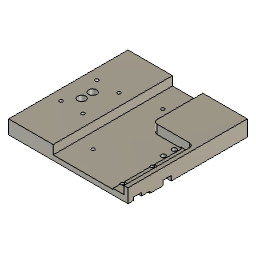
y_stage (Autodesk Fusion 360 design; units mm, degrees)
part number: 2025-09-14-19-37-15-685
Autodesk Fusion 360 part; units mm, degrees
sketch "Sketch1" plane through (0, 0, 0) normal (0, 0, 1) x (1, 0, 0)
  line L0 (-30, 30) -> (30, 30)
  line L1 (30, -30) -> (-30, -30)
  line L2 (-30, -30) -> (-30, 30)
  line L3 (-30, 30) -> (30, -30) construction
  line L4 (30, 30) -> (-30, -30) construction
  line L5 (30, -30) -> (30, 30)
  dimension "d1" = 60
  dimension "d2" = 60
  constraint horizontal L0
  constraint parallel L0 L1
  constraint coincident L3 origin
  constraint coincident L4 origin
  constraint vertical L5
  constraint horizontal L1.start L3.end
  constraint coincident L1.start L3.end
  constraint vertical L2
  measures "d1" distance of L0.start L0.end
  measures "d2" distance of L0.start L1.end
extrude "Extrude1" add sketch "Sketch1" along normal blind 8
sketch "Sketch2" plane through (0, 0, 8) normal (0, 0, 1) x (-1, 0, 0)
  line L0 (30, 30) -> (-30, 30)
  line L1 (-30, 30) -> (-30, -30)
  line L2 (-30, -30) -> (30, -30)
  line L3 (30, -30) -> (30, 30)
  line L4 (7.6, -30) -> (-7.6, -30)
  line L5 (-7.6, -30) -> (-7.6, 30)
  line L6 (-7.6, 30) -> (7.6, 30)
  line L7 (7.6, 30) -> (7.6, -30)
  line L8 (7.6, -30) -> (-7.6, 30) construction
  line L9 (-7.6, -30) -> (7.6, 30) construction
  line L10 (-7.6, 30) -> (-28, 30)
  line L11 (-28, 30) -> (-28, -5)
  line L12 (-28, -5) -> (-7.6, -5)
  line L13 (-7.6, -5) -> (-7.6, 30)
  dimension "d6" = 15.2
  dimension "d23" = 35
  dimension "d24" = 20.4
  constraint horizontal L4
  constraint perpendicular L4 L5
  constraint parallel L4 L6
  constraint parallel L5 L7
  constraint coincident L8 origin
  constraint coincident L9 origin
  constraint coincident L2 L4.start
  constraint horizontal L10
  constraint vertical L11
  constraint horizontal L12
  constraint vertical L13
  measures "d6" distance of L4.start L4.end
  measures "d23" distance of L10.end L11.end
  measures "d24" distance of L11.end L12.end
extrude "Extrude2" cut sketch "Sketch2" against normal blind 4.5 contours L0 L2 L4 L5 L6 L7 L13 | L0 L5 L10 L11 L12 L13
sketch "Sketch3" plane through (0, 0, 8) normal (0, 0, 1) x (-1, 0, 0)
  line L0 (7.6, 30) -> (-7.6, 30)
  line L1 (-7.6, 30) -> (-7.6, -30)
  line L2 (-7.6, -30) -> (7.6, -30)
  line L3 (7.6, -30) -> (7.6, 30)
  circle A0 centre (0, -17.5) radius 1.5
  circle A1 centre (0, 17.5) radius 1.5
  line L4 (7.6, 30) -> (7.6, -30)
  line L5 (7.6, -30) -> (30, -30)
  line L6 (30, -30) -> (30, 30)
  line L7 (30, 30) -> (7.6, 30)
  circle A2 centre (20.5, -2.75) radius 1.125
  circle A3 centre (20.5, 2.75) radius 1.125
  circle A4 centre (-20.5, 2.75) radius 1.125
  circle A5 centre (-20.5, -2.75) radius 1.125
  line L8 (-22.5, 11.2805) -> (-26.5, 11.2805)
  arc A6 (-26.5, 11.2805) -> (-26.5, 9.2805) centre (-26.5, 10.2805) ccw
  line L9 (-26.5, 9.2805) -> (-22.5, 9.2805)
  arc A7 (-22.5, 9.2805) -> (-22.5, 11.2805) centre (-22.5, 10.2805) ccw
  line L10 (-22.5, 10.2805) -> (-26.5, 10.2805) construction
  line L11 (-22.5, 26.2805) -> (-26.5, 26.2805)
  arc A8 (-26.5, 26.2805) -> (-26.5, 24.2805) centre (-26.5, 25.2805) ccw
  line L12 (-26.5, 24.2805) -> (-22.5, 24.2805)
  arc A9 (-22.5, 24.2805) -> (-22.5, 26.2805) centre (-22.5, 25.2805) ccw
  line L13 (-22.5, 25.2805) -> (-26.5, 25.2805) construction
  line L14 (-30, 30) -> (-30, -30)
  line L15 (-28, 30) -> (7.6, 30)
  circle A10 centre (13.6, 9) radius 1.5
  circle A11 centre (24.6, 9) radius 1.5
  circle A12 centre (13.6, -9) radius 1.5
  circle A13 centre (24.6, -9) radius 1.5
  dimension "d9" = 3
  dimension "d10" = 35
  dimension "d11" = 17.5
  dimension "d14" = 2.25
  dimension "d15" = 41
  dimension "d16" = 5.5
  dimension "d17" = 2.75
  dimension "d18" = 20.5
  dimension "d28" = 15
  dimension "d29" = 1
  dimension "d30" = 4
  dimension "d31" = 7.5
  dimension "d36" = 4.7195
  dimension "d60" = 3
  dimension "d61" = 18
  dimension "d62" = 11
  dimension "d63" = 21
  dimension "d64" = 6
  constraint equal A0 A1
  constraint vertical origin A0.centre
  constraint vertical origin A1.centre
  constraint vertical A2.centre A3.centre
  constraint horizontal A3.centre A4.centre
  constraint vertical A4.centre A5.centre
  constraint horizontal A2.centre A5.centre
  constraint equal A4 A5
  constraint equal A2 A5
  constraint equal A2 A3
  constraint tangent L8 A6
  constraint tangent A6 L9
  constraint parallel L8 L9
  constraint tangent L9 A7
  constraint tangent L8 A7
  constraint horizontal L10
  constraint tangent L11 A8
  constraint tangent A8 L12
  constraint parallel L11 L12
  constraint tangent L12 A9
  constraint tangent L11 A9
  constraint horizontal L13
  constraint vertical A7.centre A9.centre
  constraint vertical A6.centre A8.centre
  constraint equal A7 A9
  constraint horizontal A10.centre A11.centre
  constraint vertical A11.centre A13.centre
  constraint horizontal A12.centre A13.centre
  constraint vertical A10.centre A12.centre
  constraint equal A10 A12
  constraint equal A12 A13
  constraint equal A10 A11
  measures "d9" diameter of A1
  measures "d10" distance of A0.centre A1.centre
  measures "d11" distance of origin A0.centre
  measures "d14" diameter of A2
  measures "d15" distance of A2.centre A5.centre
  measures "d16" distance of A2.centre A3.centre
  measures "d17" vertical distance of origin A3.centre
  measures "d18" horizontal distance of origin A2.centre
  measures "d28" distance of A6.centre A8.centre
  measures "d29" distance of A7 L10
  measures "d30" distance of A6.end L9.end
  measures "d31" distance of A7.centre L14
  measures "d36" distance of A9.centre L15
  measures "d60" diameter of A10
  measures "d61" distance of A10.centre A12.centre
  measures "d62" distance of A10.centre A11.centre
  measures "d63" distance of L7 A11.centre
  measures "d64" distance of L3 A10.centre
extrude "Extrude3" cut sketch "Sketch3" against normal up to surface (8 mm away) contours A0 | A1 | A2 | A3 | A4 | A5 | L8 A6 L9 A7 | L11 A8 L12 A9 | A10 | A11 | A12 | A13
sketch "Sketch4" plane through (0, 0, 3.5) normal (0, 0, 1) x (-1, 0, 0)
  circle A0 centre (0, -17.5) radius 1.5
  circle A1 centre (-20.5, -2.75) radius 1.125
  circle A2 centre (0, 17.5) radius 1.5
  circle A3 centre (-20.5, 2.75) radius 1.125
  line L0 (7.6, 30) -> (-28, 30)
  line L1 (-28, 30) -> (-28, -5)
  line L2 (-28, -5) -> (-7.6, -5)
  line L3 (-7.6, -5) -> (-7.6, -30)
  line L4 (-7.6, -30) -> (7.6, -30)
  line L5 (7.6, -30) -> (7.6, 30)
  line L6 (-28, -5) -> (-22.5, -5)
  line L7 (-22.5, -5) -> (-22.5, 30)
  line L8 (-22.5, 30) -> (-28, 30)
  line L9 (-28, 30) -> (-28, -5)
  line L10 (-22.5, 24.2805) -> (-26.5, 24.2805)
  line L11 (-26.5, 26.2805) -> (-22.5, 26.2805)
  arc A4 (-22.5, 24.2805) -> (-22.5, 26.2805) centre (-22.5, 25.2805) ccw
  line L12 (-22.5, 9.2805) -> (-26.5, 9.2805)
  line L13 (-26.5, 11.2805) -> (-22.5, 11.2805)
  arc A5 (-22.5, 9.2805) -> (-22.5, 11.2805) centre (-22.5, 10.2805) ccw
  arc A6 (-26.5, 26.2805) -> (-26.5, 24.2805) centre (-26.5, 25.2805) ccw
  arc A7 (-26.5, 11.2805) -> (-26.5, 9.2805) centre (-26.5, 10.2805) ccw
  dimension "d25" = 5.5
  constraint horizontal L6
  constraint vertical L7
  constraint horizontal L8
  constraint vertical L9
  constraint coincident L0 L7.end
  constraint coincident L1.end L2.start
  measures "d25" distance of L7.end L0.end
extrude "Extrude4" add sketch "Sketch4" along normal blind 0.5 contours L0 L1 L2 L6 L7 L8 L9 L10 L11 L12 L13 A6 A7
fillet "Fillet1" radius 2 2 edges at (7.6, 5, 5.75) (28, 5, 6)
fillet "Fillet2" radius 1 1 edges at (22.5, 5, 3.75)
sketch "Sketch5" plane through (0, 0, 0) normal (0, 0, -1) x (1, 0, 0)
  circle A0 centre (20.5, 2.75) radius 1.125
  circle A1 centre (0, 17.5) radius 1
  circle A2 centre (-20.5, -2.75) radius 1.125
  line L0 (26.5, 24.2805) -> (22.5, 24.2805)
  arc A3 (22.5, 26.2805) -> (22.5, 24.2805) centre (22.5, 25.2805) ccw
  line L1 (22.5, 26.2805) -> (26.5, 26.2805)
  arc A4 (26.5, 24.2805) -> (26.5, 26.2805) centre (26.5, 25.2805) ccw
  circle A5 centre (20.5, -2.75) radius 1.125
  circle A6 centre (0, -17.5) radius 1
  circle A7 centre (-20.5, 2.75) radius 1.125
  line L2 (26.5, 9.2805) -> (22.5, 9.2805)
  arc A8 (22.5, 11.2805) -> (22.5, 9.2805) centre (22.5, 10.2805) ccw
  line L3 (22.5, 11.2805) -> (26.5, 11.2805)
  arc A9 (26.5, 9.2805) -> (26.5, 11.2805) centre (26.5, 10.2805) ccw
  line L4 (30, 30) -> (-30, 30)
  line L5 (-30, 30) -> (-30, -30)
  line L6 (-30, -30) -> (30, -30)
  line L7 (30, -30) -> (30, 30)
  line L8 (30, -30) -> (-30, -30)
  line L9 (-30, -30) -> (-30, -19.5)
  line L10 (-30, -19.5) -> (30, -19.5)
  line L11 (30, -19.5) -> (30, -30)
  line L12 (0, 0) -> (-6.6567, 0) construction
  line L13 (-30, 30) -> (-30, 19.5)
  line L14 (-30, 19.5) -> (30, 19.5)
  line L15 (30, 19.5) -> (30, 30)
  line L16 (30, 30) -> (-30, 30)
  circle A10 centre (-13.6, 9) radius 1
  circle A11 centre (-24.6, 9) radius 1
  circle A12 centre (-13.6, -9) radius 1
  circle A13 centre (-24.6, -9) radius 1
  dimension "d49" = 10.5
  constraint horizontal L8
  constraint vertical L9
  constraint horizontal L10
  constraint vertical L11
  constraint coincident L5 L9.end
  constraint coincident L6.end L7.start
  constraint coincident L12.start origin
  constraint horizontal L12
  constraint symmetric L6.end L12 L4.start
  constraint symmetric L5.end L12 L4.end
  constraint symmetric L9.end L12 L13.end
  constraint symmetric L10.end L12 L14.end
  measures "d49" distance of L5.end L9.end
extrude "Extrude5" [suppressed]
sketch "Sketch6" plane through (0, 0, 0) normal (0, 0, -1) x (1, 0, 0)
  line L0 (30, -30) -> (30, 19.5)
  line L1 (-30, 19.5) -> (-30, -30)
  line L2 (26.5, 9.2805) -> (22.5, 9.2805)
  arc A0 (22.5, 11.2805) -> (22.5, 9.2805) centre (22.5, 10.2805) ccw
  line L3 (22.5, 11.2805) -> (26.5, 11.2805)
  arc A1 (26.5, 9.2805) -> (26.5, 11.2805) centre (26.5, 10.2805) ccw
  circle A2 centre (-20.5, 2.75) radius 1.125
  circle A3 centre (0, -17.5) radius 1
  circle A4 centre (20.5, -2.75) radius 1.125
  circle A5 centre (-20.5, -2.75) radius 1.125
  circle A6 centre (0, 17.5) radius 1
  circle A7 centre (20.5, 2.75) radius 1.125
  line L4 (22.5, 23.2805) -> (26.5, 23.2805)
  arc A8 (26.5, 23.2805) -> (26.5, 27.2805) centre (26.5, 25.2805) ccw
  line L5 (26.5, 27.2805) -> (22.5, 27.2805)
  arc A9 (22.5, 27.2805) -> (22.5, 23.2805) centre (22.5, 25.2805) ccw
  line L6 (22.5, 25.2805) -> (26.5, 25.2805) construction
  line L7 (22.5, 8.2805) -> (26.5, 8.2805)
  arc A10 (26.5, 8.2805) -> (26.5, 12.2805) centre (26.5, 10.2805) ccw
  line L8 (26.5, 12.2805) -> (22.5, 12.2805)
  arc A11 (22.5, 12.2805) -> (22.5, 8.2805) centre (22.5, 10.2805) ccw
  line L9 (22.5, 10.2805) -> (26.5, 10.2805) construction
  line L10 (26.5, 27.2805) -> (30, 27.2805)
  line L11 (30, 27.2805) -> (30, 23.2805)
  line L12 (30, 23.2805) -> (26.5, 23.2805)
  line L13 (26.5, 23.2805) -> (26.5, 27.2805)
  line L14 (26.5, 12.2805) -> (30, 12.2805)
  line L15 (30, 12.2805) -> (30, 8.2805)
  line L16 (30, 8.2805) -> (26.5, 8.2805)
  line L17 (26.5, 8.2805) -> (26.5, 12.2805)
  line L18 (30, 19.5) -> (-30, 19.5)
  line L19 (-30, -30) -> (30, -30)
  circle A12 centre (-13.6, -9) radius 1
  circle A13 centre (-24.6, -9) radius 1
  circle A14 centre (-13.6, 9) radius 1
  circle A15 centre (-24.6, 9) radius 1
  arc A16 (22.5, 26.2805) -> (22.5, 24.2805) centre (22.5, 25.2805) ccw
  line L20 (26.5, 26.2805) -> (22.5, 26.2805)
  arc A17 (26.5, 24.2805) -> (26.5, 26.2805) centre (26.5, 25.2805) ccw
  line L21 (22.5, 24.2805) -> (26.5, 24.2805)
  line L22 (-30, 30) -> (-30, -30)
  line L23 (-30, -30) -> (30, -30)
  line L24 (30, -30) -> (30, 30)
  circle A18 centre (-13.6, 9) radius 1.5
  circle A19 centre (20.5, 2.75) radius 1.125
  circle A20 centre (0, 17.5) radius 1.5
  circle A21 centre (-20.5, -2.75) radius 1.125
  circle A22 centre (-24.6, 9) radius 1.5
  circle A23 centre (-13.6, -9) radius 1.5
  circle A24 centre (20.5, -2.75) radius 1.125
  circle A25 centre (0, -17.5) radius 1.5
  circle A26 centre (-20.5, 2.75) radius 1.125
  line L25 (26.5, 9.2805) -> (22.5, 9.2805)
  arc A27 (22.5, 11.2805) -> (22.5, 9.2805) centre (22.5, 10.2805) ccw
  line L26 (22.5, 11.2805) -> (26.5, 11.2805)
  arc A28 (26.5, 9.2805) -> (26.5, 11.2805) centre (26.5, 10.2805) ccw
  circle A29 centre (-24.6, -9) radius 1.5
  line L27 (26.5, 24.2805) -> (22.5, 24.2805)
  arc A30 (22.5, 26.2805) -> (22.5, 24.2805) centre (22.5, 25.2805) ccw
  line L28 (22.5, 26.2805) -> (26.5, 26.2805)
  arc A31 (26.5, 24.2805) -> (26.5, 26.2805) centre (26.5, 25.2805) ccw
  line L29 (30, 30) -> (-30, 30)
  dimension "d56" = 2
  dimension "d57" = 2
  constraint tangent L4 A8
  constraint tangent A8 L5
  constraint parallel L4 L5
  constraint tangent L5 A9
  constraint tangent L4 A9
  constraint horizontal L6
  constraint tangent L7 A10
  constraint tangent A10 L8
  constraint parallel L7 L8
  constraint tangent L8 A11
  constraint tangent L7 A11
  constraint coincident A1.centre A10.centre
  constraint parallel L4 L9
  constraint coincident A0.centre A11.centre
  constraint horizontal L10
  constraint vertical L11
  constraint horizontal L12
  constraint vertical L13
  constraint coincident L0 L11.end
  constraint collinear L4 L12
  constraint horizontal L14
  constraint vertical L15
  constraint horizontal L16
  constraint vertical L17
  constraint coincident L0 L15.end
  constraint collinear L7 L16
  constraint vertical A9.centre A0.centre
  constraint coincident A9.centre L6.start
  constraint vertical A8.centre A1.centre
  measures "d56" radius of A11
  measures "d57" radius of A9
extrude "Extrude6" cut sketch "Sketch6" against normal blind 2.5 contours L0 A10 L14 L15 L16 L24 | A1 A10 L17 A28 | L2 A0 L3 L7 L8 A11 L17 L25 A27 L26 | A8 L10 L11 L12 L24 | A8 L13 A17 A31 | L4 L5 A9 L13 A16 L20 L21 L27 A30 L28 | L13 A16 L20 L21 L27 A30 L28 | L13 A17 A31
sketch "Sketch7" plane through (0, 0, 8) normal (0, 0, 1) x (-1, 0, 0)
  circle A0 centre (13.6, 9) radius 1.5
  circle A1 centre (20.5, -2.75) radius 1.125
  circle A2 centre (24.6, 9) radius 1.5
  circle A3 centre (13.6, -9) radius 1.5
  circle A4 centre (20.5, 2.75) radius 1.125
  circle A5 centre (24.6, -9) radius 1.5
  line L0 (7.6, 30) -> (7.6, -30)
  line L1 (7.6, -30) -> (30, -30)
  line L2 (30, -30) -> (30, 30)
  line L3 (30, 30) -> (7.6, 30)
  circle A6 centre (20.5, 2.75) radius 1.125
  circle A7 centre (20.5, -2.75) radius 1.125
  circle A8 centre (20.5, 2.75) radius 2
  circle A9 centre (20.5, -2.75) radius 2
  dimension "d69" = 4
  dimension "d70" = 4
  constraint concentric A6 A8
  constraint concentric A7 A9
  measures "d69" diameter of A9
  measures "d70" diameter of A8
extrude "Extrude7" cut sketch "Sketch7" against normal up to surface (4.5 mm away) contours A8 | A9
sketch "Sketch8" plane through (-30, 0, 0) normal (-1, 0, 0) x (0, -1, 0)
  line L0 (19.5, 0) -> (19.5, 0.75)
  line L1 (19.5, 0.75) -> (30, 0.75)
  line L2 (30, 0.75) -> (30, 8)
  line L3 (30, 8) -> (-30, 8)
  line L4 (-30, 8) -> (-30, 0)
  line L5 (-30, 0) -> (19.5, 0)
  line L6 (-30, 0) -> (-22, 0)
  line L7 (-22, 0) -> (-22, 1.5)
  line L8 (-22, 1.5) -> (-30, 1.5)
  line L9 (-30, 1.5) -> (-30, 0)
  dimension "d73" = 1.5
  dimension "d74" = 8
  constraint horizontal L6
  constraint vertical L7
  constraint horizontal L8
  constraint vertical L9
  constraint coincident L4.end L5.start
  measures "d73" distance of L4.end L8.end
  measures "d74" distance of L7.end L8.end
extrude "Extrude8" [suppressed]
thread "Thread2" "ISO Metric profile 2.0 M2x0.4 M2x0.4 6H" major diameter 2.074 minor diameter 1.623 pitch 0.4 angle 60 resizes the face on face at (-1.4925, -17.3506, 2.3333) on face at (-1.4925, 17.6494, 2.3333) on face at (-26.0925, -8.8506, 2.6667) on face at (-15.0925, -8.8506, 2.6667) on face at (-26.0925, 9.1494, 2.6667) on face at (-15.0925, 9.1494, 2.6667)
sketch "Sketch10" plane through (-30, 0, 0) normal (-1, 0, 0) x (0, -1, 0)
  line L0 (-30, 0) -> (30, 0)
  line L1 (30, 0) -> (30, 8)
  line L2 (30, 8) -> (-30, 8)
  line L3 (-30, 8) -> (-30, 0)
  line L4 (30, 0) -> (19, 0)
  line L5 (19, 0) -> (19, 1)
  line L6 (19, 1) -> (30, 1)
  line L7 (30, 1) -> (30, 0)
  dimension "d88" = 1
  dimension "d90" = 11
  dimension "d97" = 49
  constraint horizontal L4
  constraint vertical L5
  constraint horizontal L6
  constraint vertical L7
  constraint coincident L0 L1.start
  measures "d88" distance of L0.end L6.end
  measures "d90" distance of L5.end L6.end
  measures "d97" distance of L0.start L4.end
extrude "Extrude10" cut sketch "Sketch10" against normal up to surface (60 mm away) contours L0 L1 L4 L5 L6 L7
sketch "Sketch9" plane through (0, 0, 8) normal (0, 0, 1) x (-1, 0, 0)
  circle A0 centre (20.28, -2.75) radius 2
  circle A1 centre (20.28, 2.75) radius 2
  circle A2 centre (13.6, 9) radius 1.5
  circle A3 centre (24.6, 9) radius 1.5
  circle A4 centre (13.6, -9) radius 1.5
  circle A5 centre (24.6, -9) radius 1.5
  line L0 (7.6, 30) -> (7.6, -30)
  line L1 (7.6, -30) -> (30, -30)
  line L2 (30, -30) -> (30, 30)
  line L3 (30, 30) -> (7.6, 30)
  line L4 (39.6, 11) -> (11.6, 11)
  line L5 (11.6, 11) -> (11.6, -11)
  line L6 (11.6, -11) -> (39.6, -11)
  line L7 (10.45, 12.5) -> (30, 12.5)
  line L8 (30, 12.5) -> (30, -12.5)
  line L9 (30, -12.5) -> (10.45, -12.5)
  line L10 (10.45, -12.5) -> (10.45, 12.5)
  dimension "d77" = 1.15
  dimension "d78" = 1.5
  dimension "d79" = 1.5
  constraint horizontal L7
  constraint vertical L8
  constraint horizontal L9
  constraint vertical L10
  constraint coincident L2 L8.end
  measures "d77" distance of L5 L10
  measures "d78" distance of L4 L7
  measures "d79" distance of L6 L9
extrude "Extrude9" [suppressed]
fillet "Fillet3" [suppressed]
equation "d2 = d1"
equation "d11 = d10 / 2"
equation "d17 = d16 / 2"
equation "d18 = d15 / 2"
equation "d36 = 6.7185275645 mm - 1.999 mm"
equation "d57 = d56"
equation "d63 = ( 60 mm - d61 ) / 2"
equation "d77 = 1.85 mm - 0.7 mm"
equation "d79 = d78"
equation "d97 = 60 mm - 11 mm"
